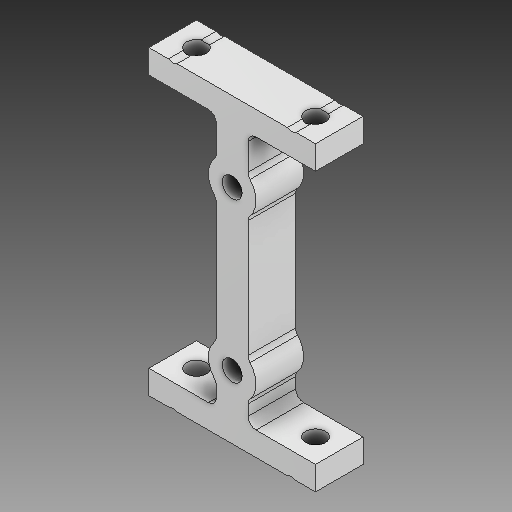
# Autodesk Inventor part: ウイング土台2
Saved by Autodesk Inventor 2020 (Build 240168000, 168)
## iProperties
Created: 2019-09-04
Part Number: ウイング土台2
Material: アルミニウム 2014-T4
Document SubType Name: Modeling
Designer: 雪村
Density: 2.8 g/cm^3
Appearance: サテン
Mass: 4.15815 g
Surface Area: 15.7688 cm^2
Volume: 1.48505 cm^3
Description: アルミ2000 6t
Author: 雪村
Autodesk Inventor part; units mm, degrees
ref_plane "YZ Plane" through (0, 0, 0) normal (1, 0, 0) x (0, 1, 0)
ref_plane "XZ Plane" through (0, 0, 0) normal (0, 1, 0) x (-1, 0, 0)
ref_plane "XY Plane" through (0, 0, 0) normal (0, 0, 1) x (1, 0, 0)
sketch "スケッチ1" plane through (0, 0, 0) normal (0, 0, 1) x (1, 0, 0)
  line L0 (0, 0) -> (21, 0)
  line L1 (0, 0) -> (0, 3)
  line L2 (21, 0) -> (21, 3)
  line L3 (21, 3) -> (12.5, 3)
  line L4 (0, 3) -> (8.5, 3)
  line L5 (0, 38) -> (21, 38)
  line L6 (0, 38) -> (0, 35)
  line L7 (21, 38) -> (21, 35)
  circle A0 centre (10.5, 28) radius 1.25
  circle A1 centre (10.5, 8) radius 1.25
  line L8 (0, 35) -> (8.5, 35)
  line L9 (21, 35) -> (12.5, 35)
  line L10 (12.5, 35) -> (12.5, 3)
  line L11 (8.5, 3) -> (8.5, 35)
  line L12 (10.5, 28) -> (10.5, 8)
  circle A2 centre (10.5, 28) radius 3
  circle A3 centre (10.5, 8) radius 3
  point P0 (10.5, 38)
  point P1 (12.5, 25.7639)
  point P2 (12.7361, 35)
  point P3 (8.2639, 35)
  point P4 (8.5, 25.7639)
  point P5 (8.5, 10.2361)
  point P6 (8.5, 5.7639)
  point P7 (12.5, 5.7639)
  point P8 (12.5, 10.2361)
  point P9 (8.5, 30.2361)
  point P10 (12.5, 30.2361)
  dimension "d0" = 21
  dimension "d1" = 21
  dimension "d2" = 38
  dimension "d3" = 2.5
  dimension "d4" = 2.5
  dimension "d5" = 20
  dimension "d6" = 10
  dimension "d7" = 2
  dimension "d8" = 2
  dimension "d9" = 3
  dimension "d10" = 3
  dimension "d11" = 6
  dimension "d12" = 6
  constraints: 26 end point, 6 vertical, 5 horizontal, 4 centre point, 3 vertical alignment, 2 coincident, 2 horizontal alignment, 1 midpoint, 1 point on line
  measures "d0" distance of L0.start L0.end
  measures "d1" distance of L5.start L5.end
  measures "d2" distance between parallel lines of L0 L5
  measures "d3" diameter of A0
  measures "d4" diameter of A1
  measures "d5" distance of L12.end L12.start
  measures "d6" distance from line of L5 L12.start
  measures "d7" distance between parallel lines of L12 L11
  measures "d8" distance between parallel lines of L10 L12
  measures "d9" distance of L5.end L7.end
  measures "d10" distance of L0.end L2.end
  measures "d11" diameter of A2
  measures "d12" diameter of A3
extrude "押し出し1" add sketch "スケッチ1" along normal blind 6
fillet "フィレット1" radius 1 12 edges at (12.5, 30.2361, 3) (12.5, 25.7639, 3) (12.5, 35, 3) (12.5, 10.2361, 3) (8.5, 25.7639, 3) (8.5, 30.2361, 3) (8.5, 10.2361, 3) (12.5, 5.7639, 3) (8.5, 5.7639, 3) (12.5, 3, 3) (8.5, 3, 3) (8.5, 35, 3)
sketch "スケッチ2" plane through (0, 0, 0) normal (0, -1, 0) x (1, 0, 0)
  line L0 (0, 0) -> (0, 6) projected
  circle A0 centre (3, 3) radius 1.25
  circle A1 centre (18, 3) radius 1.25
  point P0 (0, 3)
  dimension "d16" = 2.5
  dimension "d17" = 2.5
  dimension "d18" = 3
  dimension "d19" = 15
  constraints: 2 centre point, 2 horizontal alignment, 1 midpoint
  measures "d16" diameter of A0
  measures "d17" diameter of A1
  measures "d18" distance from line of L0 A0.centre
  measures "d19" distance of A1.centre A0.centre
extrude "押し出し2" cut sketch "スケッチ2" against normal through all
sketch "スケッチ3" plane through (0, 0, 6) normal (0, 0, 1) x (1, 0, 0)
  line L0 (1.75, 38) -> (4.25, 38) projected
  line L1 (4.25, 35) -> (1.75, 35) projected
  line L2 (16.75, 38) -> (19.25, 38) projected
  line L3 (4.25, 0) -> (1.75, 0) projected
  line L4 (19.25, 0) -> (16.75, 0) projected
  circle A0 centre (3, 38.9) radius 1.05
  circle A1 centre (18, 38.9) radius 1.05
  circle A2 centre (3, -0.9) radius 1.05
  circle A3 centre (18, -0.9) radius 1.05
  point P0 (0, 0)
  point P1 (18, 0)
  point P2 (3, 0)
  point P3 (3, 38)
  point P4 (18, 38)
  dimension "d22" = 2.1
  dimension "d23" = 2.1
  dimension "d24" = 2.1
  dimension "d25" = 2.1
  dimension "d26" = 0.9
  dimension "d27" = 0.9
  dimension "d28" = 0.9
  dimension "d29" = 0.9
  constraints: 4 centre point, 4 midpoint, 4 vertical alignment
  measures "d22" diameter of A0
  measures "d23" diameter of A1
  measures "d24" diameter of A2
  measures "d25" diameter of A3
  measures "d26" distance of point (18, 38) A1.centre
  measures "d27" distance from line of L0 A0.centre
  measures "d28" distance of point (3, 0) A2.centre
  measures "d29" distance from line of A3.centre L4
extrude "押し出し3" cut sketch "スケッチ3" against normal through all
equation "\"d1\" = d0"
equation "\"d8\" = d7"
equation "\"d27\" = d26"
equation "\"d28\" = d26"
equation "\"d29\" = d28"
